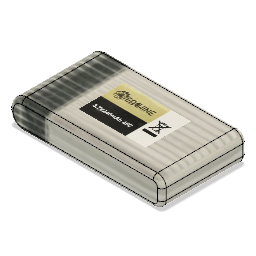
battery v1 (Autodesk Fusion 360 design; units mm, degrees)
Autodesk Fusion 360 part; units mm, degrees
sketch "Sketch1" plane through (0, 0, 0) normal (0, 1, 0) x (1, 0, 0)
  line L0 (0, 0) -> (35, 0)
  line L1 (35, 0) -> (35, -19.5)
  line L2 (35, -19.5) -> (0, -19.5)
  line L3 (0, -19.5) -> (0, 0)
  dimension "d1" = 35
  dimension "d2" = 19.5
  constraint horizontal L0
  constraint vertical L1
  constraint horizontal L2
  constraint vertical L3
  constraint coincident L0.start L3.end
  measures "d1" distance of L0.start L0.end
  measures "d2" distance of L0.start L2.end
extrude "Extrude1" add sketch "Sketch1" along normal blind 6.5 makes body 1
fillet "Fillet1" radius 3 2 edges at (0, 6.5, 9.75) (0, 0, 9.75) on bodies 1
fillet "Fillet2" radius 2 2 edges at (35, 6.5, 9.75) (35, 0, 9.75) on bodies 1
fillet "Fillet3" radius 1 16 edges at (35, 3.25, 19.5) (34.4142, 0.5858, 19.5) (18, 0, 19.5) (0.8787, 0.8787, 19.5) (0, 3.25, 19.5) (0.8787, 5.6213, 19.5) (18, 6.5, 19.5) (34.4142, 5.9142, 19.5) (0, 3.25, 0) (0.8787, 0.8787, 0) (18, 0, 0) (34.4142, 0.5858, 0) (35, 3.25, 0) (34.4142, 5.9142, 0) (18, 6.5, 0) (0.8787, 5.6213, 0) on bodies 1
copy_body "Body->Comp1" bodies 1 removing the originals makes body 2 in component "Battery"
component "Battery" placed x (1, 0, 0) y (0, 1, 0) z (0, 0, 1) at (0, 0, 0)
